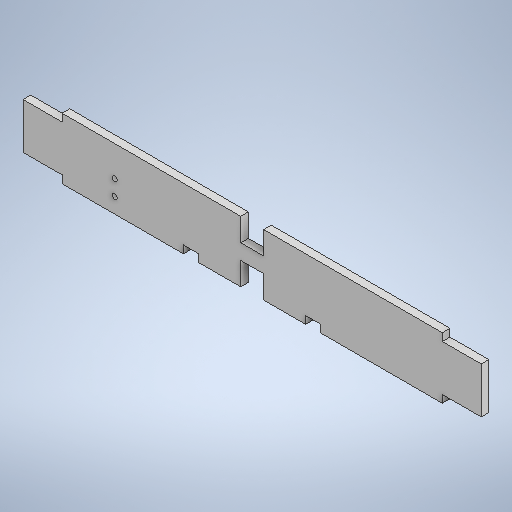
# Autodesk Inventor part: Base Leg V2 Slotted
Saved by Autodesk Inventor 2025.4 (Build 294407000, 407)
## iProperties
Created: 2026-03-23
Part Number: Base Leg V2 Slotted
Material: Generic
Document SubType Name: Sheet Metal
Designer: lenovo
Density: 1 g/cm^3
Sheet Metal Rule: Default_mm
Appearance: Default
Author: lenovo
Autodesk Inventor part; units mm, degrees
ref_plane "YZ Plane" through (0, 0, 0) normal (1, 0, 0) x (0, 1, 0)
ref_plane "XZ Plane" through (0, 0, 0) normal (0, 1, 0) x (-1, 0, 0)
ref_plane "XY Plane" through (0, 0, 0) normal (0, 0, 1) x (1, 0, 0)
sketch "Sketch1" plane through (0, 0, 0) normal (0, 0, 1) x (1, 0, 0)
  line L0 (-150, -15) -> (150, -15)
  line L1 (150, -15) -> (150, 15)
  line L2 (150, 15) -> (-150, 15)
  line L3 (-150, 15) -> (-150, -15)
  line L4 (-150, -15) -> (150, 15) construction
  line L5 (150, -15) -> (-150, 15) construction
  line L6 (-124.5, 20) -> (124.5, 20)
  line L7 (124.5, 20) -> (124.5, 15)
  line L8 (124.5, 15) -> (-124.5, 15)
  line L9 (-124.5, 15) -> (-124.5, 20)
  line L10 (-124.5, 20) -> (124.5, 15) construction
  line L11 (124.5, 20) -> (-124.5, 15) construction
  line L12 (-150, 0) -> (150, 0)
  line L13 (-124.5, -20) -> (124.5, -20)
  line L14 (124.5, -20) -> (124.5, -15)
  line L15 (124.5, -15) -> (-124.5, -15)
  line L16 (-124.5, -15) -> (-124.5, -20)
  line L17 (-124.5, -20) -> (124.5, -15) construction
  line L18 (124.5, -20) -> (-124.5, -15) construction
  point P0 (0, 0)
  point P1 (0, 0)
  point P2 (0, 17.5)
  point P3 (0, 15)
  point P4 (-77.3047, 14.0744)
  point P5 (81.6953, 14.0744)
  point P6 (0, -15)
  point P7 (0, -17.5)
  dimension "d0" = 5
  dimension "d1" = 30
  dimension "d2" = 300
  dimension "d3" = 249
  measures "d0" distance of L8.end L6.start
  measures "d1" distance of L2.end L0.start
  measures "d2" distance of L0.start L0.end
  measures "d3" distance of L6.start L6.end
extrude "Plate1" add sketch "Sketch1" along normal blind 5
sketch "Sketch3" plane through (0, 0, 5) normal (0, 0, 1) x (1, 0, 0)
  line L0 (-124.5, -20) -> (124.5, -20) projected
  line L1 (-7.5, -20) -> (7.5, -20)
  line L2 (7.5, -20) -> (7.5, -5)
  line L3 (7.5, -5) -> (-7.5, -5)
  line L4 (-7.5, -5) -> (-7.5, -20)
  point P0 (0, -5)
  point P1 (0, 0)
  dimension "d19" = 15
  constraints: 8 end point, 2 parallel, 2 perpendicular, 1 horizontal, 1 midpoint, 1 point on line, 1 vertical alignment
  measures "d19" distance of L2.end L3.end
extrude "Cut1" cut sketch "Sketch3" against normal blind 5
sketch "Sketch4" plane through (0, 0, 5) normal (0, 0, 1) x (1, 0, 0)
  circle A0 centre (-90, 0) radius 1.6
  circle A1 centre (-90, -10) radius 1.6
  line L0 (-7.5, -5) -> (7.5, -5) projected
  point P0 (0, 0)
  point P1 (0, -5)
  dimension "d9" = 3.2
  dimension "d10" = 3.2
  dimension "d12" = 10
  dimension "d21" = 90
  constraints: 2 centre point, 1 horizontal alignment, 1 midpoint, 1 vertical alignment
  measures "d9" diameter of A0
  measures "d10" diameter of A1
  measures "d12" distance of A0.centre A1.centre
  measures "d21" horizontal distance of point (0, -5) A0.centre
extrude "Cut2" cut sketch "Sketch4" against normal blind 5
sketch "Sketch5" plane through (0, 0, 5) normal (0, 0, 1) x (1, 0, 0)
  line L0 (-124.5, 20) -> (124.5, 20) projected
  line L1 (-7.5, 20) -> (7.5, 20)
  line L2 (7.5, 20) -> (7.5, 5)
  line L3 (7.5, 5) -> (-7.5, 5)
  line L4 (-7.5, 5) -> (-7.5, 20)
  line L5 (0, 20) -> (0, 0)
  dimension "d15" = 15
  constraints: 10 end point, 2 parallel, 2 perpendicular, 1 horizontal, 1 midpoint, 1 point on line, 1 vertical, 1 other
  measures "d15" distance of L2.end L3.end
extrude "Cut3" cut sketch "Sketch5" against normal blind 5
sketch "Sketch6" plane through (0, 0, 5) normal (0, 0, 1) x (1, 0, 0)
  line L0 (124.5, -20) -> (7.5, -20) projected
  line L1 (35, -20) -> (45, -20)
  line L2 (45, -20) -> (45, -15)
  line L3 (45, -15) -> (35, -15)
  line L4 (35, -15) -> (35, -20)
  line L5 (7.5, 5) -> (-7.5, 5) projected
  line L6 (0, 5) -> (0, -4.2095)
  line L7 (-35, -20) -> (-45, -20)
  line L8 (-45, -20) -> (-45, -15)
  line L9 (-45, -15) -> (-35, -15)
  line L10 (-35, -15) -> (-35, -20)
  point P0 (0, 0)
  dimension "d22" = 5
  dimension "d23" = 10
  dimension "d24" = 35
  constraints: 18 end point, 4 symmetric about line, 2 parallel, 1 horizontal, 1 midpoint, 1 perpendicular, 1 point on line, 1 vertical
  measures "d22" distance of L1.end L2.end
  measures "d23" distance of L2.end L3.end
  measures "d24" distance from line of point (0, 0) L4
extrude "Cut4" cut sketch "Sketch6" against normal blind 5
equation "\"d7\" = Thickness"
equation "\"d13\" = Thickness"
equation "\"d16\" = Thickness"
equation "\"d25\" = Thickness"
equation "\"d4\" = Thickness"
equation "\"BendRadius\" = Thickness"
equation "\"BendReliefWidth\" = Thickness"
equation "\"BendReliefDepth\" = 0.5 * Thickness"
equation "\"TransitionRadius\" = BendRadius"
equation "\"JacobiRadiusSize\" = BendRadius"
equation "\"GapSize\" = Thickness"
equation "\"Thickness\" = 5"
body "Solid1"
